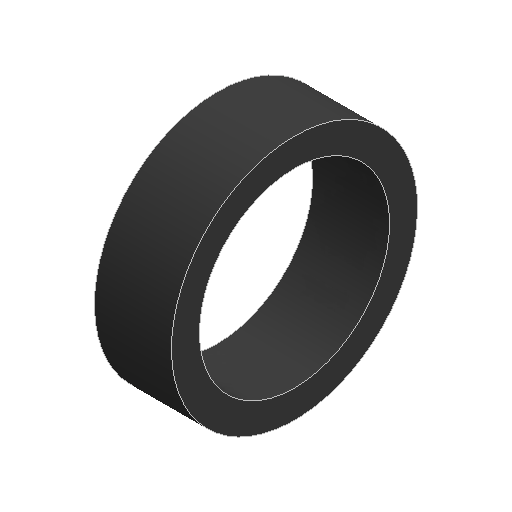
# Autodesk Inventor part: Wheel_rubber
Saved by Autodesk Inventor 2026 (Build 300175050, 175E)
## iProperties
Created: 2025-11-23
Part Number: Wheel_rubber
Material: Rubber
Document SubType Name: Modeling
Designer: Kartik
Mass: 171.652 g
Surface Area: 359.555 cm^2
Volume: 184.572 cm^3
Density: 0.93 g/cm^3
Appearance: Rubber - Black
Author: Kartik
Autodesk Inventor part; units mm, degrees
ref_plane "YZ Plane" through (0, 0, 0) normal (1, 0, 0) x (0, 1, 0)
ref_plane "XZ Plane" through (0, 0, 0) normal (0, 1, 0) x (-1, 0, 0)
ref_plane "XY Plane" through (0, 0, 0) normal (0, 0, 1) x (1, 0, 0)
sketch "Sketch1" plane through (0, 0, 0) normal (1, 0, 0) x (0, 1, 0)
  circle A0 centre (0, 0) radius 61.5
  circle A1 centre (0, 0) radius 47.5
  dimension "d0" = 123
  dimension "d3" = 14
  constraints: 2 centre point, 2 coincident
  measures "d0" diameter of A0
  measures "d3" radial gap between concentric circles of A0 A1
extrude "Extrusion1" add sketch "Sketch1" along normal blind 38.5
body "Solid1"
